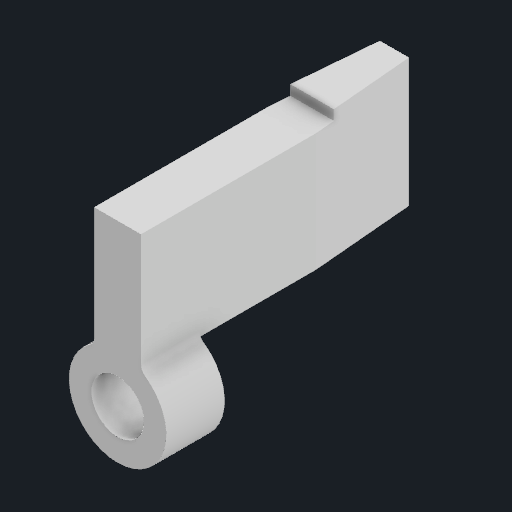
# Autodesk Inventor part: belt clip 2
Saved by Autodesk Inventor 2024.3 (Build 283343000, 343)
## iProperties
Created: 2024-09-28
Part Number: belt clip 2
Material: Generic
Document SubType Name: Modeling
Designer: MFil
Density: 1 g/cm^3
Appearance: Default
Author: MFil
Autodesk Inventor part; units mm, degrees
ref_plane "YZ Plane" through (0, 0, 0) normal (1, 0, 0) x (0, 1, 0)
ref_plane "XZ Plane" through (0, 0, 0) normal (0, 1, 0) x (-1, 0, 0)
sketch "Sketch1" plane through (0, 0, 0) normal (0, 1, 0) x (-1, 0, 0)
  line L0 (5.5341, -4.8619) -> (4.7341, -5.0029) projected
  line L1 (5.5341, -4.4619) -> (5.5341, -4.8619) projected
  line L2 (4.7341, -4) -> (5.5341, -4.4619) projected
  line L3 (4.7341, -3.0029) -> (4.7341, -4) projected
  line L4 (5.5341, -2.8619) -> (4.7341, -3.0029) projected
  line L5 (5.5341, -2.4619) -> (5.5341, -2.8619) projected
  line L6 (4.7341, -2) -> (5.5341, -2.4619) projected
  line L7 (4.7341, -1.0029) -> (4.7341, -2) projected
  line L8 (5.5341, -0.8619) -> (4.7341, -1.0029) projected
  line L9 (5.5341, -0.4619) -> (5.5341, -0.8619) projected
  line L10 (4.7341, 0) -> (5.5341, -0.4619) projected
  line L11 (10.1341, 0) -> (4.7341, 0) projected
  line L12 (9.3341, -0.4619) -> (10.1341, 0) projected
  line L13 (9.3341, -0.8619) -> (9.3341, -0.4619) projected
  line L14 (10.1341, -1.0029) -> (9.3341, -0.8619) projected
  line L15 (10.1341, -1.0029) -> (10.1341, -2) projected
  line L16 (9.3341, -2.4619) -> (10.1341, -2) projected
  line L17 (9.3341, -2.8619) -> (9.3341, -2.4619) projected
  line L18 (10.1341, -3.0029) -> (9.3341, -2.8619) projected
  line L19 (10.1341, -3.0029) -> (10.1341, -4) projected
  line L20 (9.3341, -4.4619) -> (10.1341, -4) projected
  line L21 (9.3341, -4.8619) -> (9.3341, -4.4619) projected
  line L22 (10.1341, -5.0029) -> (9.3341, -4.8619) projected
  line L23 (10.1341, -5.0029) -> (10.1341, -6) projected
  line L24 (9.3341, -6.4619) -> (10.1341, -6) projected
  line L25 (9.3341, -6.8619) -> (9.3341, -6.4619) projected
  line L26 (10.1341, -7.0029) -> (9.3341, -6.8619) projected
  line L27 (10.1341, -7.0029) -> (10.1341, -8) projected
  line L28 (9.3341, -8.4619) -> (10.1341, -8) projected
  line L29 (9.3341, -8.8619) -> (9.3341, -8.4619) projected
  line L30 (10.1336, -9.0029) -> (9.3341, -8.8619) projected
  line L31 (10.1341, -9) -> (10.1341, -10.8672) projected
  arc A0 (10.1341, -10.8672) -> (10.1663, -11.225) centre (12.1341, -10.8672) ccw projected
  line L32 (4.5189, -11.225) -> (10.1663, -11.225) projected
  arc A1 (4.5189, -11.225) -> (4.7341, -10.3226) centre (2.7341, -10.3226) ccw projected
  line L33 (4.7341, -9) -> (4.7341, -10.3226) projected
  line L34 (5.5341, -8.8619) -> (4.7346, -9.0029) projected
  line L35 (5.5341, -8.4619) -> (5.5341, -8.8619) projected
  line L36 (4.7341, -8) -> (5.5341, -8.4619) projected
  line L37 (4.7341, -7.0029) -> (4.7341, -8) projected
  line L38 (5.5341, -6.8619) -> (4.7341, -7.0029) projected
  line L39 (5.5341, -6.4619) -> (5.5341, -6.8619) projected
  line L40 (4.7341, -6) -> (5.5341, -6.4619) projected
  line L41 (4.7341, -5.0029) -> (4.7341, -6) projected
  line L42 (10.1341, 0) -> (8.6341, 0)
  line L43 (4.7341, 0) -> (6.2341, 0)
  line L44 (6.2341, 0) -> (6.2341, -6)
  line L45 (6.2341, -6) -> (8.6341, -6)
  line L46 (8.6341, -6) -> (8.6341, 0)
  line L47 (8.6341, -6) -> (8.3837, -8.8619)
  line L48 (8.6341, -6) -> (11.5069, -6) construction
  line L49 (6.2341, -6) -> (6.4845, -8.8619)
  line L50 (6.2341, -6) -> (9.1069, -6) construction
  line L51 (6.4845, -8.8619) -> (8.3837, -8.8619)
  line L52 (8.3837, -8.8619) -> (8.2259, -10.666)
  line L53 (8.2259, -10.666) -> (8.1769, -11.225)
  line L54 (6.4845, -8.8619) -> (6.6912, -11.225)
  line L55 (8.6341, 0) -> (6.2341, 0)
  line L56 (6.2341, 0) -> (6.2341, 2)
  line L57 (6.2341, 2) -> (8.6341, 2)
  line L58 (8.6341, 2) -> (8.6341, 0)
  point P0 (0, 0)
  dimension "d0" = 1.5
  dimension "d1" = 1.5
  dimension "d2" = 6
  dimension "d3" = 95
  dimension "d4" = 85
  dimension "d5" = 2
  constraints: 34 end point, 5 point on line, 4 horizontal, 4 perpendicular, 2 equal length, 2 parallel
  measures "d0" distance of L11.start L42.end
  measures "d1" distance of L10.start L43.end
  measures "d2" distance of L43.end L44.end
  measures "d3" angle of L47 L48
  measures "d4" angle of L49 L50
  measures "d5" distance of L55.end L56.end
extrude "Extrusion1" add sketch "Sketch1" against normal blind 6.6 contours L56 L57 L58 L11 | L11 L46 L45 L44 | L54 L51 L52 L53 L32 | L45 L47 L51 L49
sketch "Sketch2" plane through (-8.6341, 0, 2) normal (0, 0, 1) x (1, 0, 0)
  circle A0 centre (1.2, 2) radius 0.9
  circle A1 centre (1.2, -8.8) radius 0.9
  circle A2 centre (1.2, 2) radius 2.5
  circle A3 centre (1.2, -8.8) radius 2.5
  line L0 (0, 0) -> (2.4, 0) projected
  line L1 (0, 0) -> (0, -6.6) projected
  line L2 (2.4, -6.6) -> (0, -6.6) projected
  line L3 (2.4, 0) -> (2.4, -6.6) projected
  line L4 (2.4, 0) -> (2.4, -6.6) projected
  line L5 (2.4, -6.6) -> (2.4, -6.4)
  line L6 (2.4, -6.4) -> (2.4, -6.087)
  line L7 (0, -6.4) -> (0, -6.0348)
  circle A4 centre (2.9, -6.3282) radius 0.5
  circle A5 centre (-0.5, -6.3282) radius 0.5
  line L8 (0, 0) -> (0, -6.6) projected
  circle A6 centre (1.2, -8.8) radius 1.1 projected
  circle A7 centre (1.2, 2) radius 1.1 projected
  line L9 (3.9, 0.2) -> (3.9, -6.8) projected
  line L10 (3.9, -6.8) -> (-1.5, -6.8) projected
  line L11 (-1.5, -6.8) -> (-1.5, 0.2) projected
  line L12 (-1.5, 0.2) -> (3.9, 0.2) projected
  line L13 (-8, -25.631) -> (-8, 3.869) projected
  line L14 (8.6341, -25.631) -> (-8, -25.631) projected
  line L15 (8.6341, -25.631) -> (8.6341, 3.869) projected
  line L16 (-8, 3.869) -> (8.6341, 3.869) projected
  point P0 (8.6341, 0)
  point P1 (0, -6.3282)
  point P2 (-0.2167, -6.7401)
  point P3 (2.6167, -6.7401)
  point P4 (2.4, -6.3282)
  point P5 (2.4, -0.1932)
  point P6 (0, -0.1932)
  dimension "d16" = 5
  dimension "d17" = 5
  dimension "d19" = 0.2
  dimension "d20" = 1
  dimension "d21" = 1
  constraints: 6 centre point, 6 end point, 4 coincident, 4 point on line, 4 tangent, 2 vertical alignment, 1 concentric, 1 other
  measures "d16" diameter of A3
  measures "d17" diameter of A2
  measures "d19" distance of L2.start L5.end
  measures "d20" diameter of A4
  measures "d21" diameter of A5
ref_plane "Work Plane1" through (-16.6341, -25.631, 0) normal (0, 0, 1) x (1, 0, 0)
extrude "Extrusion3" add sketch "Sketch2" along normal blind 1 and the other way blind 2 contours A0 | A1 | A2 L12 L16 | L16 A2 | A2 L3 L0 L1 L12 | L3 L2 A3 L1 A2 | A2 L1 L0 L3 | A4 A3 L2 L3 | L1 L2 A3 A5 | A3 L10 L2 | A3 L10 | L2 A3 | A6 | A7
sketch "Sketch3" plane through (-8.6341, 0, 3) normal (0, 0, 1) x (1, 0, 0)
  circle A0 centre (1.2, -8.8) radius 0.9 projected
  circle A1 centre (1.2, 2) radius 0.9 projected
  point P0 (8.6341, 0)
fillet "Fillet1" radius 0.6 1 edges at (-6.2341, -0.1932, 1.5)
hole "Hole1" at (-7.4341, -8.8, 3) at (-7.4341, 2, 3) direction (0, 0, -1) diameter 2.7 end through all clearance for "Countersunk Flat Head Screw ISO 2009/7046" size "M2.5" standard "ISO"
sketch "Sketch4" plane through (-8.6341, 0, 3) normal (0, 0, 1) x (1, 0, 0)
  arc A0 (2.6516, -0.0354) -> (2.4, -0.5239) centre (3, -0.5239) ccw projected
  line L0 (3, -0.5239) -> (-1.7059, -0.5239)
  line L1 (-1.7059, -0.5239) -> (-1.7059, 4.8856)
  line L2 (-1.7059, 4.8856) -> (3, 4.8856)
  line L3 (3, 4.8856) -> (3, -0.5239)
  line L4 (3, -0.5239) -> (6.6824, -0.5239)
  line L5 (6.6824, -0.5239) -> (6.6824, 3.9617)
  line L6 (6.6824, 3.9617) -> (3, 3.9617)
  line L7 (3, 3.9617) -> (3, -0.5239)
  point P0 (8.6341, 0)
  constraints: 16 end point, 4 parallel, 2 horizontal, 2 perpendicular
extrude "Extrusion4" cut sketch "Sketch4" against normal blind 10
body "Solid1"
